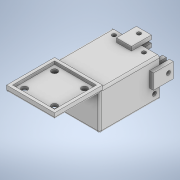
# Autodesk Inventor part: carriageEndR
Saved by Autodesk Inventor 2020 (Build 240168000, 168)
## iProperties
Created: 2020-01-10
Part Number: carriageEndR
Material: Generic
Document SubType Name: Modeling
Designer: PAB
Density: 1 g/cm^3
Appearance: Default
Author: PAB
Autodesk Inventor part; units mm, degrees
ref_plane "YZ Plane" through (0, 0, 0) normal (1, 0, 0) x (0, 1, 0)
ref_plane "XZ Plane" through (0, 0, 0) normal (0, 1, 0) x (-1, 0, 0)
ref_plane "XY Plane" through (0, 0, 0) normal (0, 0, 1) x (1, 0, 0)
sketch "Sketch1" plane through (0, 0, 0) normal (0, 1, 0) x (-1, 0, 0)
  line L0 (24, 138) -> (-24, 138)
  line L1 (-24, 138) -> (-24, -138)
  line L2 (-24, -138) -> (24, -138)
  line L3 (24, -138) -> (24, 138)
  point P0 (0, 0)
  dimension "d0" = 48
  dimension "d1" = 276
  constraints: 8 end point, 2 parallel, 1 horizontal, 1 perpendicular
  measures "d0" distance of L2.end L1.end
  measures "d1" distance of L1.end L0.end
extrude "Extrusion1" add sketch "Sketch1" along normal blind 3
sketch "Sketch2" plane through (0, 3, 0) normal (0, 1, 0) x (1, 0, 0)
  line L0 (-24, 138) -> (-24, -138) projected
  line L1 (-24, -138) -> (-21, -138)
  line L2 (-21, -138) -> (-21, -90)
  line L3 (-21, -90) -> (-24, -90)
  line L4 (-24, -90) -> (-24, -138)
  line L5 (24, -138) -> (24, 138) projected
  line L6 (-21, -90) -> (24, -90)
  line L7 (24, -90) -> (24, -93)
  line L8 (24, -93) -> (-21, -93)
  line L9 (-21, -93) -> (-21, -90)
  line L10 (-24, -138) -> (24, -138) projected
  line L11 (24, -93) -> (21, -93)
  line L12 (21, -93) -> (21, -138)
  line L13 (21, -138) -> (24, -138)
  line L14 (24, -138) -> (24, -93)
  line L15 (21, -138) -> (-21, -138)
  line L16 (-21, -138) -> (-21, -135)
  line L17 (-21, -135) -> (21, -135)
  line L18 (21, -135) -> (21, -138)
  point P0 (0, 0)
  dimension "d4" = 3
  dimension "d5" = 48
  dimension "d6" = 3
  dimension "d7" = 3
  dimension "d8" = 3
  constraints: 32 end point, 8 parallel, 4 horizontal, 4 perpendicular, 3 point on line
  measures "d4" distance of L3.end L2.end
  measures "d5" distance of L2.end L1.end
  measures "d6" distance of L6.end L7.end
  measures "d7" distance of L13.end L12.end
  measures "d8" distance of L15.end L16.end
extrude "Extrusion2" add sketch "Sketch2" along normal blind 3 contours L3 L2 L1 L0 | L6 L5 L8 L2 | L2 L17 L12 L10 | L12 L8 L5 L10
mirror "Mirror1" about plane through (0, 0, 0) normal (0, 0, 1) of "Extrusion2"
sketch "Sketch3" plane through (0, 0, 0) normal (0, -1, 0) x (1, 0, 0)
  line L0 (24, -90) -> (-24, -90) projected
  line L1 (24, 138) -> (24, -138) projected
  line L2 (-24, -90) -> (24, -90)
  line L3 (24, -90) -> (24, -93)
  line L4 (24, -93) -> (-24, -93)
  line L5 (-24, -93) -> (-24, -90)
  line L6 (-24, 90) -> (24, 90) projected
  line L7 (24, 90) -> (21, 90)
  line L8 (21, 90) -> (21, -90)
  line L9 (21, -90) -> (24, -90)
  line L10 (24, -90) -> (24, 90)
  line L11 (-24, 90) -> (24, 90)
  line L12 (24, 90) -> (24, 93)
  line L13 (24, 93) -> (-24, 93)
  line L14 (-24, 93) -> (-24, 90)
  point P0 (0, 0)
  dimension "d11" = 3
  dimension "d12" = 3
  dimension "d13" = 3
  constraints: 24 end point, 6 parallel, 3 horizontal, 3 perpendicular, 3 point on line
  measures "d11" distance of L2.end L3.end
  measures "d12" distance of L9.end L8.end
  measures "d13" distance of L12.end L11.end
extrude "Extrusion3" add sketch "Sketch3" along normal blind 35
sketch "Sketch4" plane through (-24, 0, -90) normal (0, 0, 1) x (1, 0, 0)
  line L0 (0, -35) -> (45, -35) projected
  line L1 (45, 0) -> (45, -35) projected
  line L2 (0, -35) -> (45, -35)
  line L3 (45, -35) -> (45, -31)
  line L4 (45, -31) -> (0, -31)
  line L5 (0, -31) -> (0, -35)
  point P0 (24, 0)
  dimension "d16" = 4
  constraints: 8 end point, 2 parallel, 1 horizontal, 1 perpendicular, 1 point on line
  measures "d16" distance of L3.end L2.end
extrude "Extrusion4" add sketch "Sketch4" along normal blind 8
sketch "Sketch5" plane through (-24, -31, -90) normal (0, 1, 0) x (1, 0, 0)
  line L0 (0, -8) -> (45, -8) projected
  line L1 (45, 0) -> (45, -8) projected
  line L2 (0, -8) -> (45, -8)
  line L3 (45, -8) -> (45, -4)
  line L4 (45, -4) -> (0, -4)
  line L5 (0, -4) -> (0, -8)
  point P0 (24, -90)
  dimension "d19" = 4
  constraints: 8 end point, 2 parallel, 1 horizontal, 1 midpoint, 1 perpendicular
  measures "d19" distance of L3.end L2.end
extrude "Extrusion5" add sketch "Sketch5" along normal blind 4
sketch "Sketch6" plane through (0, 0, 0) normal (0, -1, 0) x (1, 0, 0)
  line L0 (21, -86) -> (-24, -86) projected
  line L1 (-24, -82) -> (21, -82)
  line L2 (21, -82) -> (21, -86)
  line L3 (21, -86) -> (-24, -86)
  line L4 (-24, -86) -> (-24, -82)
  point P0 (0, 0)
  dimension "d22" = 4
  constraints: 8 end point, 2 parallel, 1 horizontal, 1 perpendicular
  measures "d22" distance of L1.end L0.start
extrude "Extrusion6" add sketch "Sketch6" along normal blind 4
mirror "Mirror2" about plane through (0, 0, 0) normal (0, 0, 1) of "Extrusion6", "Extrusion5", "Extrusion4"
sketch "Sketch7" plane through (0, 0, 0) normal (0, -1, 0) x (1, 0, 0)
  circle A0 centre (-15, -129) radius 3
  circle A1 centre (15, -129) radius 3
  circle A2 centre (15, -99) radius 3
  circle A3 centre (-15, -99) radius 3
  point P0 (0, 0)
  dimension "d25" = 6
  dimension "d26" = 6
  dimension "d27" = 6
  dimension "d28" = 6
  constraints: 4 centre point
  measures "d25" diameter of A0
  measures "d26" diameter of A1
  measures "d27" diameter of A2
  measures "d28" diameter of A3
extrude "Extrusion7" cut sketch "Sketch7" against normal blind 4
mirror "Mirror3" about plane through (0, 0, 0) normal (0, 0, 1) of "Extrusion7"
sketch "Sketch8" plane through (0, 0, 0) normal (0, -1, 0) x (1, 0, 0)
  line L0 (21, 82) -> (21, -82) projected
  line L1 (-24, -82) -> (-24, 82) projected
  line L2 (21, -20) -> (-24, -20)
  line L3 (-24, -20) -> (-24, -17)
  line L4 (-24, -17) -> (21, -17)
  line L5 (21, -17) -> (21, -20)
  point P0 (0, 0)
  dimension "d31" = 3
  constraints: 8 end point, 2 parallel, 2 point on line, 1 horizontal, 1 perpendicular
  measures "d31" distance of L2.end L3.end
extrude "Extrusion8" add sketch "Sketch8" along normal blind 42.3
sketch "Sketch9" plane through (21, 0, -20) normal (0, 0, -1) x (-1, 0, 0)
  circle A0 centre (39.35, -5.65) radius 4
  circle A1 centre (39.35, -36.65) radius 4
  circle A2 centre (8.35, -5.65) radius 4
  circle A3 centre (8.35, -36.65) radius 4
  point P0 (21, 0)
  dimension "d34" = 8
  dimension "d35" = 8
  dimension "d36" = 8
  dimension "d37" = 8
  constraints: 4 centre point
  measures "d34" diameter of A0
  measures "d35" diameter of A1
  measures "d36" diameter of A2
  measures "d37" diameter of A3
extrude "Extrusion9" add sketch "Sketch9" along normal blind 3
sketch "Sketch10" plane through (-18.35, -36.65, -23) normal (0, 0, -1) x (-1, 0, 0)
  circle A0 centre (0, 0) radius 3
  circle A1 centre (0, 31) radius 4 projected
  circle A2 centre (0, 31) radius 3
  circle A3 centre (-31, 0) radius 4 projected
  circle A4 centre (-31, 0) radius 3
  circle A5 centre (-31, 31) radius 4 projected
  circle A6 centre (-31, 31) radius 3
  point P0 (-18.35, 36.65)
  dimension "d40" = 6
  dimension "d41" = 6
  dimension "d42" = 6
  dimension "d43" = 6
  constraints: 4 centre point, 3 coincident
  measures "d40" diameter of A0
  measures "d41" diameter of A2
  measures "d42" diameter of A4
  measures "d43" diameter of A6
extrude "Extrusion10" cut sketch "Sketch10" against normal blind 2 contours A0 | A2 | A4 | A6
sketch "Sketch11" plane through (21, 0, -20) normal (0, 0, -1) x (-1, 0, 0)
  circle A0 centre (23.85, -21.15) radius 12.5
  circle A1 centre (39.35, -36.65) radius 3 projected
  circle A2 centre (39.35, -36.65) radius 2
  circle A3 centre (8.35, -36.65) radius 3 projected
  circle A4 centre (8.35, -36.65) radius 2
  circle A5 centre (8.35, -5.65) radius 4 projected
  circle A6 centre (8.35, -5.65) radius 2
  circle A7 centre (39.35, -5.65) radius 4 projected
  circle A8 centre (39.35, -5.65) radius 2
  point P0 (21, 0)
  dimension "d46" = 25
  dimension "d47" = 4
  dimension "d48" = 4
  dimension "d49" = 4
  dimension "d50" = 4
  constraints: 5 centre point, 4 coincident
  measures "d46" diameter of A0
  measures "d47" diameter of A2
  measures "d48" diameter of A4
  measures "d49" diameter of A6
  measures "d50" diameter of A8
extrude "Extrusion11" cut sketch "Sketch11" along normal mid plane 10 contours A0 | A2 | A4 | A6 | A8
sketch "Sketch12" plane through (0, 0, 0) normal (0, -1, 0) x (1, 0, 0)
  line L0 (-24, -17) -> (-24, 82) projected
  line L1 (-24, 33) -> (24, 33)
  line L2 (24, 33) -> (24, -138)
  line L3 (24, -138) -> (-24, -138)
  line L4 (-24, -138) -> (-24, 33)
  point P0 (0, 0)
  constraints: 8 end point, 2 parallel, 1 horizontal, 1 perpendicular, 1 point on line
extrude "Extrusion12" cut sketch "Sketch12" along normal mid plane 100
sketch "Sketch13" plane through (0, 0, 0) normal (0, -1, 0) x (1, 0, 0)
  line L0 (-9, 43) -> (6, 43)
  line L1 (6, 43) -> (6, 23)
  line L2 (6, 23) -> (-9, 23)
  line L3 (-9, 23) -> (-9, 43)
  point P0 (0, 0)
  dimension "d55" = 15
  dimension "d56" = 20
  constraints: 8 end point, 2 parallel, 1 horizontal, 1 perpendicular
  measures "d55" distance of L1.end L2.end
  measures "d56" distance of L0.end L1.end
extrude "Extrusion13" add sketch "Sketch13" along normal blind 4 and the other way blind 7
sketch "Sketch14" plane through (21, 0, 86) normal (-1, 0, 0) x (0, 0, 1)
  line L0 (-43, -20) -> (-63, -20)
  line L1 (-63, -20) -> (-63, -5)
  line L2 (-63, -5) -> (-43, -5)
  line L3 (-43, -5) -> (-43, -20)
  point P0 (-86, 0)
  dimension "d61" = 20
  dimension "d62" = 15
  constraints: 8 end point, 2 parallel, 1 horizontal, 1 perpendicular
  measures "d61" distance of L1.end L2.end
  measures "d62" distance of L0.end L1.end
extrude "Extrusion14" add sketch "Sketch14" along normal blind 4 and the other way blind 7
sketch "Sketch15" plane through (21, 0, 86) normal (-1, 0, 0) x (0, 0, 1)
  circle A0 centre (-58, -12.5) radius 2
  circle A1 centre (-48, -27.5) radius 2
  point P0 (-86, 0)
  dimension "d67" = 4
  dimension "d68" = 4
  constraints: 2 centre point
  measures "d67" diameter of A0
  measures "d68" diameter of A1
extrude "Extrusion15" cut sketch "Sketch15" along normal mid plane 20
sketch "Sketch16" plane through (0, 0, 0) normal (0, -1, 0) x (1, 0, 0)
  circle A0 centre (-16.5, 38) radius 2
  circle A1 centre (-1.5, 28) radius 2
  circle A2 centre (13.5, 38) radius 2
  point P0 (0, 0)
  dimension "d71" = 4
  dimension "d72" = 4
  dimension "d73" = 4
  constraints: 3 centre point
  measures "d71" diameter of A0
  measures "d72" diameter of A1
  measures "d73" diameter of A2
extrude "Extrusion16" cut sketch "Sketch16" along normal mid plane 20
sketch "Sketch17" plane through (6, -4, 23) normal (0, 0, -1) x (-1, 0, 0)
  line L0 (-18, 7) -> (0, 7) projected
  line L1 (15, 4) -> (15, 0) projected
  line L2 (0, 7) -> (15, 7)
  line L3 (15, 7) -> (15, 4)
  line L4 (15, 4) -> (0, 4)
  line L5 (0, 4) -> (0, 7)
  line L6 (-15, -16) -> (-18, -16)
  line L7 (-18, -16) -> (-18, -1)
  line L8 (-18, -1) -> (-15, -1)
  line L9 (-15, -1) -> (-15, -16)
  point P0 (6, 4)
  dimension "d76" = 3
  constraints: 16 end point, 4 parallel, 2 horizontal, 2 perpendicular
  measures "d76" distance of L2.end L1.start
extrude "Extrusion17" cut sketch "Sketch17" against normal blind 10
fillet "Fillet1" radius 2 8 edges at (-24, 0, 115.5) (0, 0, 138) (24, 0, 115.5) (0, -35, 93) (-24, 3, 61.5) (24, -35, 63) (24, 3, 61.5) (24, -17.5, 93)
body "Solid1"
